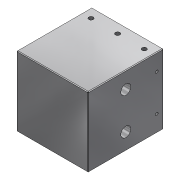
# Autodesk Inventor part: BC-10002
Saved by Autodesk Inventor 2016 (Build 200138000, 138)
## iProperties
Created: 2015-11-16
Part Number: BC-10002
Project: DIPOLO BC - 3T SIRIUS
Cost Center: 1504002005
Material: Aço Carbono AISI 1006
Document SubType Name: Modeling
Designer: reinaldo.basilio
Mass: 9825.23 g
Surface Area: 794.75 cm^2
Volume: 1248.44 cm^3
Density: 7.87 g/cm^3
Appearance: Silver
Description: Base de fechamento magnético dos blocos central.
RuleStatus: InUse
AfterMaterialChange0: file://_iMaterial
AfterAnyiPropertyChange0: file://_iMaterial
AfterDocNew0: file://_Naming_par
AfterDocNew1: file://_NameStart
AfterDocNew2: file://_NameStart1
AfterDocNew3: file://_Materiais
DocNumber: XXXXX-XXX-XXXX-00-001.ipt
Folder: .
Title: DIPOLO BC - 3T SIRIUS
Author: reinaldo.basilio
Subject: BC-10002
Autodesk Inventor part; units mm, degrees
ref_plane "YZ Plane" through (0, 0, 0) normal (1, 0, 0) x (0, 1, 0)
ref_plane "XZ Plane" through (0, 0, 0) normal (0, 1, 0) x (-1, 0, 0)
ref_plane "XY Plane" through (0, 0, 0) normal (0, 0, 1) x (1, 0, 0)
sketch "Sketch5" plane through (0, 0, 0) normal (0, 1, 0) x (-1, 0, 0)
  line L0 (56.5, 52.5) -> (-56.5, 52.5)
  line L1 (-56.5, 52.5) -> (-56.5, -52.5)
  line L2 (-56.5, -52.5) -> (56.5, -52.5)
  line L3 (56.5, -52.5) -> (56.5, 52.5)
  point P0 (0, 0)
  point P1 (56.5, 0)
  point P2 (0, 52.5)
  dimension "d8" = 113
  dimension "d9" = 105
  constraints: 8 end point, 2 midpoint, 2 parallel, 1 horizontal, 1 horizontal alignment, 1 perpendicular, 1 vertical alignment
  measures "d8" distance of L0.start L0.end
  measures "d9" distance of L0.end L1.end
extrude "Extrusion5" add sketch "Sketch5" along normal blind 107.5
sketch "Sketch8" plane through (0, 107.5, 0) normal (0, 1, 0) x (1, 0, 0)
  circle A0 centre (0, 27.5) radius 7
  circle A1 centre (0, -27.5) radius 7
  line L0 (-56.5, -52.5) -> (56.5, -52.5) projected
  line L1 (56.5, -52.5) -> (56.5, 52.5) projected
  line L2 (56.5, 52.5) -> (-56.5, 52.5) projected
  line L3 (-56.5, 52.5) -> (-56.5, -52.5) projected
  point P0 (0, 52.5)
  point P1 (0, -52.5)
  point P2 (56.5, 0)
  point P3 (-56.5, 0)
  point P4 (0, -52.5)
  dimension "d21" = 113
  dimension "d22" = 105
  dimension "d61" = 55
  dimension "d62" = 27.5
  constraints: 5 midpoint, 3 vertical alignment, 2 centre point, 1 equal radius, 1 horizontal alignment
  measures "d21" distance of L0.start L0.end
  measures "d22" distance of L2.end L0.start
  measures "d61" distance of A0.centre A1.centre
  measures "d62" vertical distance of point (-56.5, 0) A1.centre
hole "Hole1" at (0, 107.5, 27.5) at (0, 107.5, -27.5) direction (0, -1, 0) diameter 9 end through all counterbore diameter 15 counterbore depth 45 clearance for "Socket Head Cap Screw" size "M8" standard "Ansi Metric M Profile"
sketch "Sketch9" plane through (-56.5, 0, 52.5) normal (0, 0, 1) x (1, 0, 0)
  line L0 (0, 0) -> (0, 107.5) projected
  circle A0 centre (15, 93.75) radius 4
  circle A1 centre (15, 53.75) radius 4
  circle A2 centre (15, 13.75) radius 4
  point P0 (113, 0)
  point P1 (113, 107.5)
  point P2 (56.5, 0)
  point P3 (0, 53.75)
  dimension "d36" = 107.5
  dimension "d37" = 40
  dimension "d38" = 40
  dimension "d40" = 8
  dimension "d41" = 15
  constraints: 3 centre point, 2 equal radius, 2 vertical alignment, 1 horizontal alignment, 1 midpoint
  measures "d36" distance of point (113, 107.5) point (113, 0)
  measures "d37" distance of A0.centre A1.centre
  measures "d38" distance of A2.centre A1.centre
  measures "d40" diameter of A0
  measures "d41" distance from line of L0 A0.centre
hole "Hole2" at (-41.5, 93.75, 52.5) at (-41.5, 53.75, 52.5) at (-41.5, 13.75, 52.5) direction (0, 0, -1) diameter 6.647 depth 15 tip angle 118 thread size "M8x1.25" class "6H" standard "ISO Metric profile"
sketch "Sketch10" plane through (56.5, 0, -52.5) normal (0, 0, -1) x (-1, 0, 0)
  circle A0 centre (98, 93.75) radius 4
  circle A1 centre (98, 53.75) radius 4
  circle A2 centre (98, 13.75) radius 4
  circle A3 centre (98, 53.75) radius 3.3235 projected
  circle A4 centre (98, 13.75) radius 3.3235 projected
  circle A5 centre (98, 93.75) radius 3.3235 projected
  dimension "d52" = 8
  constraints: 3 centre point, 3 concentric, 2 equal radius, 2 vertical alignment
  measures "d52" diameter of A0
hole "Hole3" at (-41.5, 93.75, -52.5) at (-41.5, 53.75, -52.5) at (-41.5, 13.75, -52.5) direction (0, 0, 1) diameter 6.647 depth 15 tip angle 118 thread size "M8x1.25" class "6H" standard "ISO Metric profile"
sketch "Sketch11" plane through (0, 107.5, 0) normal (0, 1, 0) x (1, 0, 0)
  line L0 (-56.5, 52.5) -> (-56.5, -52.5) projected
  circle A0 centre (-46.5, -27.5) radius 4
  circle A1 centre (-46.5, 27.5) radius 4
  point P0 (0, 0)
  dimension "d63" = 55
  dimension "d64" = 10
  dimension "d65" = 8
  dimension "d73" = 27.5
  constraints: 2 centre point, 1 equal radius, 1 vertical alignment
  measures "d63" distance of A1.centre A0.centre
  measures "d64" distance from line of A0.centre L0
  measures "d65" diameter of A0
  measures "d73" vertical distance of point (0, 0) A1.centre
hole "Hole4" at (-46.5, 107.5, 27.5) at (-46.5, 107.5, -27.5) direction (0, -1, 0) diameter 4.134 depth 15 tip angle 118 thread size "M5x0.8" class "6H" standard "ISO Metric profile"
chamfer "Chamfer2" distance 1 angle 45 12 edges at (56.5, 53.75, -52.5) (56.5, 53.75, 52.5) (-56.5, 53.75, 52.5) (-56.5, 53.75, -52.5) (0, 107.5, -52.5) (-56.5, 107.5, 0) (0, 107.5, 52.5) (56.5, 107.5, 0) (0, 0, -52.5) (-56.5, 0, 0) (0, 0, 52.5) (56.5, 0, 0)
equation "\"d62\" = 0.5 * d61"
equation "\"d38\" = d37"
equation "\"d73\" = 0.5 * d63"
body "Solid5"
